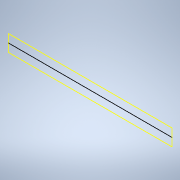
# Autodesk Inventor part: leg_bone_1
Saved by Autodesk Inventor 2020 (Build 240168000, 168)
## iProperties
Created: 2019-05-01
Part Number: leg_bone_1
Material: Generic
Document SubType Name: Modeling
Designer: psrob
Density: 1 g/cm^3
Appearance: Default
Author: psrob
Autodesk Inventor part; units mm, degrees
ref_plane "YZ Plane" through (0, 0, 0) normal (1, 0, 0) x (0, 1, 0)
ref_plane "XZ Plane" through (0, 0, 0) normal (0, 1, 0) x (-1, 0, 0)
ref_plane "XY Plane" through (0, 0, 0) normal (0, 0, 1) x (1, 0, 0)
sketch "Sketch1" plane through (0, 0, 0) normal (0, 0, 1) x (1, 0, 0)
  line L0 (0, -1) -> (0, -9) projected
  line L1 (0, -9) -> (50, -9) projected
  line L2 (50, -1) -> (50, -9) projected
  line L3 (0, -1) -> (50, -1) projected
  line L4 (50, -5) -> (0, -5)
  line L5 (25, -5) -> (-15, -5)
  circle A0 centre (-15, -5) radius 8
  line L6 (-15, -5) -> (-15, -13)
  line L7 (-15, -5) -> (-15, 3)
  line L8 (-15, -13) -> (0, -13)
  line L9 (0, -13) -> (0, 3)
  line L10 (0, 3) -> (-15, 3)
  line L11 (-15, 3) -> (-15, -13)
  line L12 (0, -13) -> (15, -13)
  line L13 (15, -13) -> (15, 3)
  line L14 (15, 3) -> (0, 3)
  line L15 (0, 3) -> (0, -13)
  dimension "d0" = 40
  dimension "d1" = 16
  dimension "d2" = 15
  dimension "d3" = 16
  dimension "d4" = 15
  dimension "d5" = 16
  constraints: 24 end point, 4 parallel, 3 midpoint, 2 horizontal, 2 perpendicular, 2 point on circle, 1 centre point, 1 coincident, 1 point on line, 1 vertical
  measures "d0" distance of L5.start L5.end
  measures "d1" diameter of A0
  measures "d2" distance of L10.end L9.end
  measures "d3" distance of L9.end L8.end
  measures "d4" distance of L14.end L13.end
  measures "d5" distance of L13.end L12.end
extrude "Extrusion1" add sketch "Sketch1" along normal blind 4 contours L3 L13 L4 L0 | L9 L14 L13 L3 | L0 L5 A0 L10 L9 | L4 L13 L1 L0 | L0 L9 L8 A0 L5 | L1 L13 L12 L9 | A0 L6 L5 | L5 L7 A0 | L7 L6 A0
body "Solid1"
